Autodesk Inventor part; units mm, degrees
(part 2 of 2)
sketch "Sketch18" plane through (0, 0, -0.2) normal (0, 0, -1) x (-1, 0, 0)
  line L0 (-13.9597, 17.5749) -> (-9.7521, 15.1456) projected
  line L1 (-9.7521, 15.1456) -> (-5.5444, 17.5749) projected
  line L2 (-5.5444, 17.5749) -> (-5.5444, 22.4335) projected
  line L3 (-5.5444, 22.4335) -> (-9.7521, 24.8628) projected
  line L4 (-9.7521, 24.8628) -> (-13.9597, 22.4335) projected
  line L5 (-13.9597, 22.4335) -> (-13.9597, 17.5749) projected
  line L6 (-34.8886, 65.4022) -> (-34.8886, 72.3894) projected
  line L7 (-34.8886, 72.3894) -> (-40.9397, 75.883) projected
  line L8 (-40.9397, 75.883) -> (-46.9908, 72.3894) projected
  line L9 (-46.9908, 72.3894) -> (-46.9908, 65.4022) projected
  line L10 (-46.9908, 65.4022) -> (-40.9397, 61.9086) projected
  line L11 (-40.9397, 61.9086) -> (-34.8886, 65.4022) projected
  line L12 (-49.5403, 66.4665) -> (-49.5403, 71.3251) projected
  line L13 (-49.5403, 71.3251) -> (-53.7479, 73.7544) projected
  line L14 (-53.7479, 73.7544) -> (-57.9556, 71.3251) projected
  line L15 (-57.9556, 71.3251) -> (-57.9556, 66.4665) projected
  line L16 (-57.9556, 66.4665) -> (-53.7479, 64.0372) projected
  line L17 (-53.7479, 64.0372) -> (-49.5403, 66.4665) projected
  line L18 (0, 0) -> (-63.5, 0)
  line L19 (-63.5, 0) -> (-63.5, 88.9)
  line L20 (-63.5, 88.9) -> (0, 88.9)
  line L21 (0, 88.9) -> (0, 0)
  line L22 (-40.9397, 26.9914) -> (-46.9908, 23.4978) projected
  line L23 (-46.9908, 23.4978) -> (-46.9908, 16.5106) projected
  line L24 (-46.9908, 16.5106) -> (-40.9397, 13.017) projected
  line L25 (-40.9397, 13.017) -> (-34.8886, 16.5106) projected
  line L26 (-34.8886, 16.5106) -> (-34.8886, 23.4978) projected
  line L27 (-34.8886, 23.4978) -> (-40.9397, 26.9914) projected
  line L28 (-22.5603, 13.017) -> (-16.5092, 16.5106) projected
  line L29 (-16.5092, 16.5106) -> (-16.5092, 23.4978) projected
  line L30 (-16.5092, 23.4978) -> (-22.5603, 26.9914) projected
  line L31 (-22.5603, 26.9914) -> (-28.6114, 23.4978) projected
  line L32 (-28.6114, 23.4978) -> (-28.6114, 16.5106) projected
  line L33 (-28.6114, 16.5106) -> (-22.5603, 13.017) projected
  line L34 (-24.4329, 66.1976) -> (-24.4329, 72.4542) projected
  line L35 (-22.5603, 61.9086) -> (-16.5092, 65.4022) projected
  line L36 (-16.5092, 65.4022) -> (-16.5092, 72.3894) projected
  line L37 (-16.5092, 72.3894) -> (-22.5603, 75.883) projected
  line L38 (-22.5603, 75.883) -> (-28.6114, 72.3894) projected
  line L39 (-28.6114, 72.3894) -> (-28.6114, 65.4022) projected
  line L40 (-28.6114, 65.4022) -> (-22.5603, 61.9086) projected
  line L41 (-34.8886, 40.9564) -> (-34.8886, 47.9436) projected
  line L42 (-34.8886, 47.9436) -> (-40.9397, 51.4372) projected
  line L43 (-40.9397, 51.4372) -> (-46.9908, 47.9436) projected
  line L44 (-46.9908, 47.9436) -> (-46.9908, 40.9564) projected
  line L45 (-46.9908, 40.9564) -> (-40.9397, 37.4628) projected
  line L46 (-40.9397, 37.4628) -> (-34.8886, 40.9564) projected
  line L47 (-28.6114, 47.9436) -> (-28.6114, 40.9564) projected
  line L48 (-22.5603, 37.4628) -> (-16.5092, 40.9564) projected
  line L49 (-16.5092, 40.9564) -> (-16.5092, 47.9436) projected
  line L50 (-16.5092, 47.9436) -> (-22.5603, 51.4372) projected
  line L51 (-22.5603, 51.4372) -> (-28.6114, 47.9436) projected
  line L52 (-28.6114, 40.9564) -> (-22.5603, 37.4628) projected
  spline S0 degree 2 poles (-51.7802, 78.7192) (-51.7802, 77.55) (-52.7929, 76.3809) (-53.6162, 76.3809) knots 0 0 0 0.5 1 1 1 projected
  spline S1 degree 2 poles (-53.6162, 76.3809) (-53.9702, 76.3809) (-54.596, 76.6361) (-54.8841, 76.9572) knots 0 0 0 0.5 1 1 1 projected
  spline S2 degree 2 poles (-54.8841, 76.9572) (-55.197, 77.2948) (-55.6087, 78.5874) (-55.6087, 79.6413) knots 0 0 0 0.5 1 1 1 projected
  spline S3 degree 2 poles (-55.6087, 79.6413) (-55.6087, 79.8554) (-55.5922, 80.1353) (-55.584, 80.2835) knots 0 0 0 0.5 1 1 1 projected
  spline S4 degree 2 poles (-55.584, 80.2835) (-55.1476, 80.5552) (-54.2502, 80.8434) (-53.7726, 80.8434) knots 0 0 0 0.5 1 1 1 projected
  spline S5 degree 2 poles (-53.7726, 80.8434) (-53.4186, 80.8434) (-52.7435, 80.7034) (-52.4718, 80.4894) knots 0 0 0 0.5 1 1 1 projected
  spline S6 degree 2 poles (-52.4718, 80.4894) (-52.1095, 80.193) (-51.7802, 79.3449) (-51.7802, 78.7192) knots 0 0 0 0.5 1 1 1 projected
  spline S7 degree 2 poles (-51.352, 76.2245) (-50.9157, 76.6691) (-50.397, 77.9946) (-50.397, 78.7768) knots 0 0 0 0.5 1 1 1 projected
  spline S8 degree 2 poles (-50.397, 78.7768) (-50.397, 79.6496) (-50.9404, 80.9504) (-51.5002, 81.3703) knots 0 0 0 0.5 1 1 1 projected
  spline S9 degree 2 poles (-51.5002, 81.3703) (-51.986, 81.7326) (-52.8752, 81.9714) (-53.468, 81.9714) knots 0 0 0 0.5 1 1 1 projected
  spline S10 degree 2 poles (-53.468, 81.9714) (-54.0773, 81.9714) (-55.0982, 81.6009) (-55.584, 81.2633) knots 0 0 0 0.5 1 1 1 projected
  spline S11 degree 2 poles (-55.584, 81.2633) (-55.4358, 82.9429) (-53.8797, 84.6555) (-52.6117, 84.6555) knots 0 0 0 0.5 1 1 1 projected
  spline S12 degree 2 poles (-52.6117, 84.6555) (-52.2165, 84.6555) (-51.5249, 84.4826) (-51.3356, 84.3838) knots 0 0 0 0.5 1 1 1 projected
  line L53 (-51.3356, 84.3838) -> (-51.2779, 84.3838) projected
  line L54 (-51.2779, 84.3838) -> (-51.2779, 85.6929) projected
  spline S13 degree 2 poles (-51.2779, 85.6929) (-51.5002, 85.767) (-52.093, 85.8328) (-52.4306, 85.8328) knots 0 0 0 0.5 1 1 1 projected
  spline S14 degree 2 poles (-52.4306, 85.8328) (-53.575, 85.8328) (-55.3205, 84.9683) (-55.8722, 84.1944) knots 0 0 0 0.5 1 1 1 projected
  spline S15 degree 2 poles (-55.8722, 84.1944) (-56.4403, 83.404) (-56.9837, 81.2715) (-56.9837, 79.946) knots 0 0 0 0.5 1 1 1 projected
  spline S16 degree 2 poles (-56.9837, 79.946) (-56.9837, 78.5957) (-56.3909, 76.7432) (-55.8639, 76.1915) knots 0 0 0 0.5 1 1 1 projected
  spline S17 degree 2 poles (-55.8639, 76.1915) (-55.4358, 75.7305) (-54.3078, 75.2694) (-53.6244, 75.2694) knots 0 0 0 0.5 1 1 1 projected
  spline S18 degree 2 poles (-53.6244, 75.2694) (-52.9411, 75.2694) (-51.8049, 75.7552) (-51.352, 76.2245) knots 0 0 0 0.5 1 1 1 projected
  spline S19 degree 2 poles (-11.7198, 10.5254) (-11.7198, 11.6945) (-10.7071, 12.8637) (-9.8838, 12.8637) knots 0 0 0 0.5 1 1 1 projected
  spline S20 degree 2 poles (-9.8838, 12.8637) (-9.5298, 12.8637) (-8.904, 12.6084) (-8.6159, 12.2873) knots 0 0 0 0.5 1 1 1 projected
  spline S21 degree 2 poles (-8.6159, 12.2873) (-8.303, 11.9498) (-7.8913, 10.6571) (-7.8913, 9.6033) knots 0 0 0 0.5 1 1 1 projected
  spline S22 degree 2 poles (-7.8913, 9.6033) (-7.8913, 9.3892) (-7.9078, 9.1092) (-7.916, 8.961) knots 0 0 0 0.5 1 1 1 projected
  spline S23 degree 2 poles (-7.916, 8.961) (-8.3524, 8.6893) (-9.2498, 8.4012) (-9.7274, 8.4012) knots 0 0 0 0.5 1 1 1 projected
  spline S24 degree 2 poles (-9.7274, 8.4012) (-10.0814, 8.4012) (-10.7565, 8.5411) (-11.0282, 8.7552) knots 0 0 0 0.5 1 1 1 projected
  spline S25 degree 2 poles (-11.0282, 8.7552) (-11.3905, 9.0516) (-11.7198, 9.8997) (-11.7198, 10.5254) knots 0 0 0 0.5 1 1 1 projected
  spline S26 degree 2 poles (-12.148, 13.0201) (-12.5843, 12.5755) (-13.103, 11.2499) (-13.103, 10.4678) knots 0 0 0 0.5 1 1 1 projected
  spline S27 degree 2 poles (-13.103, 10.4678) (-13.103, 9.595) (-12.5596, 8.2941) (-11.9998, 7.8742) knots 0 0 0 0.5 1 1 1 projected
  spline S28 degree 2 poles (-11.9998, 7.8742) (-11.514, 7.512) (-10.6248, 7.2732) (-10.032, 7.2732) knots 0 0 0 0.5 1 1 1 projected
  spline S29 degree 2 poles (-10.032, 7.2732) (-9.4227, 7.2732) (-8.4018, 7.6437) (-7.916, 7.9813) knots 0 0 0 0.5 1 1 1 projected
  spline S30 degree 2 poles (-7.916, 7.9813) (-8.0642, 6.3017) (-9.6203, 4.5891) (-10.8883, 4.5891) knots 0 0 0 0.5 1 1 1 projected
  spline S31 degree 2 poles (-10.8883, 4.5891) (-11.2835, 4.5891) (-11.9751, 4.762) (-12.1644, 4.8608) knots 0 0 0 0.5 1 1 1 projected
  line L55 (-12.1644, 4.8608) -> (-12.2221, 4.8608) projected
  line L56 (-12.2221, 4.8608) -> (-12.2221, 3.5517) projected
  spline S32 degree 2 poles (-12.2221, 3.5517) (-11.9998, 3.4776) (-11.407, 3.4117) (-11.0694, 3.4117) knots 0 0 0 0.5 1 1 1 projected
  spline S33 degree 2 poles (-11.0694, 3.4117) (-9.925, 3.4117) (-8.1795, 4.2763) (-7.6278, 5.0502) knots 0 0 0 0.5 1 1 1 projected
  spline S34 degree 2 poles (-7.6278, 5.0502) (-7.0597, 5.8406) (-6.5163, 7.973) (-6.5163, 9.2986) knots 0 0 0 0.5 1 1 1 projected
  spline S35 degree 2 poles (-6.5163, 9.2986) (-6.5163, 10.6489) (-7.1091, 12.5014) (-7.6361, 13.053) knots 0 0 0 0.5 1 1 1 projected
  spline S36 degree 2 poles (-7.6361, 13.053) (-8.0642, 13.5141) (-9.1922, 13.9752) (-9.8756, 13.9752) knots 0 0 0 0.5 1 1 1 projected
  spline S37 degree 2 poles (-9.8756, 13.9752) (-10.5589, 13.9752) (-11.6951, 13.4894) (-12.148, 13.0201) knots 0 0 0 0.5 1 1 1 projected
  constraints: 8 end point, 2 parallel, 1 horizontal, 1 perpendicular, 38 other
extrude "Extrusion21" add sketch "Sketch18" along normal blind 0.4 bodies 3
fillet "Fillet2" radius 3.175 8 edges at (63.5, 0, 0.2) (63.5, 88.9, 0.2) (0, 0, 0.2) (0, 88.9, 0.2) (63.5, 0, -0.3) (63.5, 88.9, -0.3) (0, 0, -0.3) (0, 88.9, -0.3)
